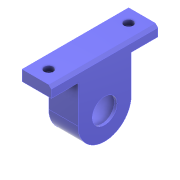
# Autodesk Inventor part: bearing holder
Saved by Autodesk Inventor 2022 (Build 260153000, 153)
## iProperties
Created: 2024-03-20
Part Number: bearing holder
Material: Generic
Document SubType Name: Modeling
Designer: david
Density: 1 g/cm^3
Appearance: Smooth - Dark Forest Green
Author: david
Autodesk Inventor part; units mm, degrees
ref_plane "YZ Plane" through (0, 0, 0) normal (1, 0, 0) x (0, 1, 0)
ref_plane "XZ Plane" through (0, 0, 0) normal (0, 1, 0) x (-1, 0, 0)
ref_plane "XY Plane" through (0, 0, 0) normal (0, 0, 1) x (1, 0, 0)
sketch "Sketch1" plane through (0, 0, 0) normal (1, 0, 0) x (0, 1, 0)
  line L0 (0, 0) -> (14, 0) construction
  line L1 (0, -10) -> (14, -10)
  line L2 (14, 10) -> (0, 10)
  arc A0 (0, 10) -> (0, -10) centre (0, 0) ccw
  arc A1 (14, -10) -> (14, 10) centre (14, 0) ccw construction
  line L3 (14, 10) -> (14, -10)
  point P0 (7, 0)
  dimension "d2" = 20
  dimension "d1" = 14
  constraints: 10 end point, 4 point on circle, 4 tangent, 2 centre point, 1 horizontal, 1 midpoint, 1 parallel, 1 vertical
  measures "d2" diameter of A1
  measures "d1" distance from line of L0.start L3
extrude "Extrusion1" add sketch "Sketch1" along normal mid plane 10
sketch "Sketch2" plane through (-5, 14, 10) normal (0, 1, 0) x (1, 0, 0)
  line L0 (0, -10) -> (10, -10)
  line L1 (10, -10) -> (10, 30)
  line L2 (10, 30) -> (0, 30)
  line L3 (0, 30) -> (0, -10)
  line L4 (0, 0) -> (0, 20) construction
  line L5 (0, 20) -> (10, 20) construction
  line L6 (10, 20) -> (10, 0) construction
  line L7 (10, 0) -> (0, 0) construction
  line L8 (0, 0) -> (0, 20) construction
  line L9 (10, 20) -> (10, 0) construction
  line L10 (0, 10) -> (10, 10) construction
  point P0 (5, 10)
  dimension "d28" = 40
  constraints: 10 end point, 2 collinear, 2 midpoint, 2 parallel, 1 horizontal, 1 perpendicular, 1 other
  measures "d28" distance between parallel lines of L2 L0
extrude "Extrusion2" add sketch "Sketch2" along normal blind 4
sketch "Sketch3" plane through (-5, 14, 10) normal (0, -1, 0) x (1, 0, 0)
  line L0 (10, -30) -> (0, -30) projected
  line L1 (0, -30) -> (0, -20) projected
  line L2 (0, -20) -> (0, 0) projected
  line L3 (0, 0) -> (0, 10) projected
  line L4 (0, 10) -> (10, 10) projected
  line L5 (10, 10) -> (10, 0) projected
  line L6 (10, 0) -> (10, -20) projected
  line L7 (10, -20) -> (10, -30) projected
  line L8 (10, -20) -> (0, -20) projected
  line L9 (0, 0) -> (10, 0) projected
  line L10 (0, 10) -> (10, 10) projected
  point P0 (5, -10)
  point P1 (5, 5)
  point P2 (5, -25)
  point P3 (5, 10)
  point P4 (5, 10)
  point P5 (5, 10)
  dimension "d30" = 5
  dimension "d31" = 5
  constraints: 4 vertical alignment, 3 midpoint
  measures "d30" distance from line of L0 point (5, -25)
  measures "d31" distance from line of point (5, 5) L4
hole "Hole1" at (0, 14, 15) at (0, 14, -15) direction (0, 1, 0) diameter 3.4 end through all counterbore diameter 6 counterbore depth 2
sketch "Sketch5" plane through (5, 0, 0) normal (1, 0, 0) x (0, 0, -1)
  arc A0 (-10, 0) -> (10, 0) centre (0, 0) ccw projected
  constraints: 1 coincident
hole "Hole3" at (5, 0, 0) direction (-1, 0, 0) diameter 13 end through all
thicken "Thicken1" operation add thickness 0.15 both sides no extend neighbours yes toward (0, 0.0804666, -0.9967573) faces at (1.6667, 0.523, -6.4789)
sketch "Sketch6" plane through (5, 0, 0) normal (1, 0, 0) x (0, 0, -1)
  circle A0 centre (0, 0) radius 6.65 construction
  line L0 (20, 18) -> (20, 14) projected
  line L1 (20, 14) -> (10, 14) projected
  line L2 (10, 14) -> (10, 0) projected
  arc A1 (-10, 0) -> (10, 0) centre (0, 0) ccw projected
  line L3 (-10, 0) -> (-10, 14) projected
  line L4 (-10, 14) -> (-20, 14) projected
  line L5 (-20, 14) -> (-20, 18) projected
  line L6 (-20, 18) -> (20, 18) projected
  circle A2 centre (0, 0) radius 6.65 projected
  line L7 (20, 18) -> (20, 14) projected
  line L8 (20, 14) -> (10, 14) projected
  line L9 (10, 14) -> (10, 0) projected
  arc A3 (-10, 0) -> (10, 0) centre (0, 0) ccw projected
  line L10 (-10, 0) -> (-10, 14) projected
  line L11 (-10, 14) -> (-20, 14) projected
  line L12 (-20, 14) -> (-20, 18) projected
  line L13 (-20, 18) -> (20, 18) projected
  circle A4 centre (0, 0) radius 4.65
  dimension "d37" = 2
  constraints: 1 centre point
  measures "d37" radial gap between concentric circles of A0 A4
extrude "Extrusion3" add sketch "Sketch6" along normal blind 1 contours L0 L1 L2 A1 L3 L4 L5 L6 | A2
chamfer "Chamfer2" distance 0.5 angle 45 1 edges at (-5, 0, 6.65)
chamfer "Chamfer3" distance 1 angle 45 1 edges at (6, 18, 0)
equation "\"d31\" = d30"
equation "\"d21\" = diameter"
equation "\"diameter\" = 13"
body "Solid1"
